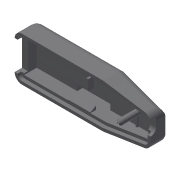
# Autodesk Inventor part: enclbase
Saved by Autodesk Inventor 2022 Beta2 (Build 260130000, 130) ContinuousBuild 0
## iProperties
Shininess: 64.0
Length Units: 11269
Angle Units: 11279
Time Units: 11290
Mass Units: 11283
Length Display Precision: 3
Angle Display Precision: 2
Created: 2002-02-13
Part Number: enclbase
Document SubType Name: Modeling
Designer: Administrator
Density: 1 g/cm^3
Material: Generic
Appearance: Light Gray
Density: 0.0
Volumn: 0.0
Area: 0.0
PropertySet Name: Model Information
Control State: 0
Master: False
Checked Out: False
Last Check In By: PMILLER
Last Check In Date: 2007-04-03
Author: Administrator
Autodesk Inventor part; units mm, degrees
sketch "Sketch1" plane through (0, 0, 0) normal (0, 0, 1) x (1, 0, 0)
  line L0 (8.2169, 11.6469) -> (8.2169, -7.4031)
  line L1 (8.2169, -7.4031) -> (46.3169, -7.4031)
  line L2 (46.3169, -7.4031) -> (66.9544, -4.2281)
  line L3 (66.9544, -4.2281) -> (66.9544, 8.4719)
  line L4 (66.9544, 8.4719) -> (46.3169, 11.6469)
  line L5 (46.3169, 11.6469) -> (8.2169, 11.6469)
  line L6 (66.9544, 2.1219) -> (8.2169, 2.1219) construction
  dimension "d0" = 19.05
  dimension "d1" = 38.1
  dimension "d2" = 58.7375
  dimension "d3" = 12.7
  constraints: 14 end point, 2 equal length, 2 midpoint, 2 parallel, 1 horizontal, 1 perpendicular, 1 vertical
  measures "d0" distance of L0.start L0.end
  measures "d1" distance of L4.end L0.start
  measures "d2" horizontal distance of L3.end L0.start
  measures "d3" distance of L2.end L3.end
extrude "Extrusion1" add sketch "Sketch1" along normal blind 9.525
sketch "Sketch2" plane through (8.2169, -7.4031, 0) normal (0, -1, 0) x (1, 0, 0)
  line L0 (38.1, 0) -> (38.1, 9.525) projected
  line L1 (38.1, 0) -> (58.7375, 0)
  line L2 (58.7375, 0) -> (58.7375, 3.175)
  line L3 (58.7375, 3.175) -> (38.1, 0)
  line L4 (58.7375, 9.525) -> (38.1, 9.525) projected
  line L5 (58.7375, 0) -> (58.7375, 9.525) projected
  dimension "d6" = 6.35
  constraints: 6 end point, 2 perpendicular, 1 collinear
  measures "d6" distance from line of L4 L2.end
extrude "Extrusion2" cut sketch "Sketch2" against normal through all contours L3 L2 L1
shell "Shell1" thickness 2.54 removed faces 1 at (20.9169, -1.0531, 9.525)
sketch "Sketch3" plane through (0, 0, 9.525) normal (0, 0, 1) x (1, 0, 0)
  line L0 (64.4144, 6.2927) -> (64.4144, -2.049) projected
  line L1 (64.4144, -2.049) -> (46.1226, -4.8631) projected
  line L2 (46.1226, -4.8631) -> (10.7569, -4.8631) projected
  line L3 (10.7569, -4.8631) -> (10.7569, 9.1069) projected
  line L4 (10.7569, 9.1069) -> (46.1226, 9.1069) projected
  line L5 (46.1226, 9.1069) -> (64.4144, 6.2927) projected
  line L6 (66.9544, -4.2281) -> (46.3169, -7.4031) projected
  line L7 (66.9544, 8.4719) -> (66.9544, -4.2281) projected
  line L8 (9.4869, 10.3769) -> (46.2197, 10.3769)
  line L9 (46.2197, 10.3769) -> (65.6844, 7.3823)
  line L10 (65.6844, 7.3823) -> (65.6844, -3.1386)
  line L11 (65.6844, -3.1386) -> (46.2197, -6.1331)
  line L12 (46.2197, -6.1331) -> (9.4869, -6.1331)
  line L13 (9.4869, -6.1331) -> (9.4869, 10.3769)
  dimension "d10" = 1.27
  dimension "d11" = 1.27
  dimension "d12" = 1.27
  dimension "d13" = 1.27
  dimension "d14" = 1.27
  constraints: 12 end point, 4 parallel, 3 perpendicular
  measures "d10" horizontal distance of L3.end L8.start
  measures "d11" horizontal distance of L2.end L12.end
  measures "d12" horizontal distance of L9.end L0.start
  measures "d13" distance between parallel lines of L9 L5
  measures "d14" distance from line of L0.end L11
extrude "Extrusion3" cut sketch "Sketch3" against normal blind 1.5875
fillet "Fillet1" radius 3.175 11 edges at (8.2169, 11.6469, 4.7625) (8.2169, -7.4031, 4.7625) (8.2169, 2.1219, 0) (27.2669, -7.4031, 0) (46.3169, -7.4031, 4.7625) (56.6356, -5.8156, 1.5875) (66.9544, -4.2281, 6.35) (27.2669, 11.6469, 0) (46.3169, 11.6469, 4.7625) (56.6356, 10.0594, 1.5875) (66.9544, 8.4719, 6.35)
fillet "Fillet2" radius 1.5875 4 edges at (9.4869, 10.3769, 8.7313) (9.4869, -6.1331, 8.7313) (65.6844, 7.3823, 8.7313) (65.6844, -3.1386, 8.7313)
ref_plane "Work Plane1" through (23.4569, -4.8631, 2.54) normal (1, 0, 0) x (0, 0, -1)
sketch "Sketch4" plane through (66.9544, -1.5043, 9.525) normal (1, 0, 0) x (0, 0, -1)
  line L0 (6.35, 0.4142) -> (6.35, 6.838) projected
  line L1 (2.3812, 8.8028) -> (0, 8.8028)
  line L2 (0, 8.8028) -> (0, 2.4528)
  line L3 (0, 2.4528) -> (0, 2.4528)
  line L4 (2.3812, 4.834) -> (2.3812, 8.8028)
  line L5 (0, -3.1381) -> (3.6261, -3.1381) projected
  line L6 (1.5875, 7.5246) -> (1.5875, -0.2724) projected
  line L7 (0, 7.2522) -> (0, 0) projected
  arc A0 (0, 2.4528) -> (2.3812, 4.834) centre (0, 4.834) ccw
  ellipse E0 centre (3.1376, 6.7638) end of major axis (5.4352, 9.0613) minor radius 3.175 (6.35, 6.838) -> (6.3231, 7.2522) ccw projected
  line L8 (0, 7.2522) -> (6.3231, 7.2522) projected
  line L9 (6.3231, 0) -> (0, 0) projected
  ellipse E1 centre (3.1376, 0.4885) end of major axis (5.4352, -1.8091) minor radius 3.175 (6.3231, 0) -> (6.35, 0.4142) ccw projected
  line L10 (3.6261, 10.3903) -> (0, 10.3903) projected
  point P0 (2.3813, 2.4528)
  dimension "d20" = 6.35
  dimension "d21" = 2.3813
  dimension "d63" = 2.3813
  dimension "d78" = 1.5875
  constraints: 8 end point, 2 perpendicular, 2 point on circle, 2 point on line, 2 tangent, 1 centre point, 1 collinear, 1 parallel, 1 vertical, 2 other
  measures "d20" distance of L1.end L2.end
  measures "d21" distance of L2.end point (2.381, 2.453)
  measures "d63" radius of A0
  measures "d78" distance between parallel lines of L10 L1
extrude "Extrusion4" cut sketch "Sketch4" against normal up to surface (43.4975 mm away) contours L8 L2 L1 L4 | L4 A0 L6 L8 | A0 L2 L8 L6
sketch "Sketch5" plane through (8.2169, -4.2281, 3.175) normal (-1, 0, 0) x (0, 0, 1)
  line L0 (0, 12.7) -> (6.35, 12.7) projected
  line L1 (3.175, 12.7) -> (6.35, 12.7)
  line L2 (6.35, 12.7) -> (6.35, 0)
  line L3 (6.35, 0) -> (3.175, 0)
  line L4 (3.175, 0) -> (3.175, 12.7)
  line L5 (4.7625, -0.3175) -> (4.7625, 13.0175) projected
  line L6 (6.35, 0) -> (6.35, 12.7) projected
  dimension "d26" = 3.175
  constraints: 8 end point, 2 collinear, 2 parallel, 1 horizontal, 1 perpendicular
  measures "d26" distance of L2.end L3.end
extrude "Extrusion5" cut sketch "Sketch5" against normal up to surface (15.24 mm away)
ref_plane "Work Plane2" through (0, 0, 4.7625) normal (0, 0, 1) x (1, 0, 0)
sketch "Sketch6" plane through (0, 0, 4.7625) normal (0, 0, 1) x (1, 0, 0)
  line L0 (55.6831, 7.636) -> (55.6831, -3.3923)
  line L1 (56.4769, 7.5139) -> (56.4769, -3.2702)
  line L2 (64.4144, -2.049) -> (64.4144, 2.5014) projected
  line L3 (57.8767, -3.0548) -> (46.1226, -4.8631) projected
  line L4 (46.1226, 9.1069) -> (64.4144, 6.2927) projected
  line L5 (55.6831, -3.3923) -> (56.4769, -3.2702)
  line L6 (56.4769, 7.5139) -> (55.6831, 7.636)
  dimension "d31" = 0.7937
  dimension "d32" = 7.9375
  constraints: 8 end point, 2 collinear, 1 parallel, 1 vertical
  measures "d31" distance between parallel lines of L1 L0
  measures "d32" distance between parallel lines of L2 L1
extrude "Extrusion6" add sketch "Sketch6" against normal up to next
ref_plane "Work Plane3" through (0, 0, 12.7) normal (0, 0, 1) x (1, 0, 0)
sketch "Sketch7" plane through (0, 0, 12.7) normal (0, 0, 1) x (1, 0, 0)
  circle A0 centre (56.08, 2.1219) radius 1.1906
  circle A1 centre (56.08, 2.1219) radius 5.3897 construction
  circle A2 centre (56.08, 2.1219) radius 0.3969 construction
  line L0 (57.8767, -3.0548) -> (46.1226, -4.8631) projected
  line L1 (46.1226, 9.1069) -> (64.4144, 6.2927) projected
  line L2 (56.4769, -3.2702) -> (56.4769, 7.5139) projected
  line L3 (55.6831, 7.636) -> (55.6831, -3.3923) projected
  dimension "d36" = 2.3813
  constraints: 4 tangent, 3 centre point, 2 coincident
  measures "d36" diameter of A0
extrude "Extrusion7" add sketch "Sketch7" against normal up to surface contours A0 L2 | L2 A0 L3 | L3 A0 surface through (66.5681, -7.4031, 5.6855) normal (-0.1520572, 0, 0.9883717)
sketch "Sketch8" plane through (56.08, 2.1219, 12.7) normal (0, 0, 1) x (1, 0, 0)
  circle A0 centre (0, 0) radius 1.1906 projected
  circle A1 centre (0, 0) radius 0.3969
  dimension "d39" = 0.7937
  constraints: 1 centre point, 1 coincident
  measures "d39" diameter of A1
extrude "Extrusion8" cut sketch "Sketch8" against normal up to surface contours A1 surface through (66.5681, -7.4031, 5.6855) normal (-0.1520572, 0, 0.9883717)
sketch "Sketch10" plane through (10.7569, -4.8631, 2.54) normal (0, 0, 1) x (1, 0, 0)
  line L0 (0, 13.97) -> (0, 0) projected
  line L1 (17.4625, 13.97) -> (31.75, 13.97)
  line L2 (31.75, 13.97) -> (31.75, 11.5887)
  line L3 (17.4625, 11.5887) -> (17.4625, 13.97)
  line L4 (17.4625, 11.5887) -> (31.75, 11.5887)
  dimension "d48" = 2.3813
  dimension "d49" = 14.2875
  dimension "d50" = 17.4625
  constraints: 8 end point, 2 parallel, 1 horizontal, 1 perpendicular
  measures "d48" distance of L3.start L1.start
  measures "d49" distance of L2.end L3.start
  measures "d50" distance from line of L1.start L0
extrude "Extrusion10" cut sketch "Sketch10" against normal up to surface (2.54 mm away)
ref_plane "Work Plane4" through (56.08, 2.1219, 12.7) normal (0, -1, 0) x (1, 0, 0)
chamfer "Chamfer1" distance 0.7937 angle 45 1 edges at (54.8894, 2.1219, 12.7)
ref_plane "Work Plane5" through (34.5694, 6.7256, 2.54) normal (1, 0, 0) x (0, 0, -1)
sketch "Sketch12" plane through (34.5694, 6.7256, 2.54) normal (1, 0, 0) x (0, 0, -1)
  line L0 (-5.3975, 2.3813) -> (-5.3975, 2.1273)
  line L1 (-5.3975, 2.1273) -> (-3.0162, 0.7938)
  line L2 (-3.0162, 0.7938) -> (-3.0162, 2.3813)
  line L3 (-3.0162, 2.3813) -> (-5.3975, 2.3813)
  line L4 (-5.3975, 2.3813) -> (-5.3975, 1.7463) projected
  line L5 (0, 2.3813) -> (-5.3975, 2.3813) projected
  dimension "d67" = 1.5875
  dimension "d68" = 2.3813
  dimension "d69" = 0.254
  constraints: 8 end point, 2 collinear, 1 parallel, 1 perpendicular, 1 vertical
  measures "d67" distance of L1.end L2.end
  measures "d68" distance of L2.end L0.start
  measures "d69" distance of L0.start L0.end
extrude "Extrusion12" add sketch "Sketch12" along normal mid plane 9.525
mirror "Mirror1" about plane through (56.08, 2.1219, 12.7) normal (0, -1, 0) of "Extrusion10", "Extrusion12"
sketch "Sketch13" plane through (46.1226, -4.8631, 2.54) normal (0, 0, 1) x (1, 0, 0)
  line L0 (-3.6158, 11.5887) -> (-17.9033, 11.5888) projected
  line L1 (-17.9033, 11.5888) -> (-17.9033, 13.97) projected
  line L2 (-17.9033, 2.3813) -> (-3.6158, 2.3813) projected
  line L3 (-11.5533, 9.2075) -> (-10.7595, 9.2075)
  line L4 (-10.7595, 9.2075) -> (-10.7595, 4.7625)
  line L5 (-10.7595, 4.7625) -> (-11.5533, 4.7625)
  line L6 (-11.5533, 4.7625) -> (-11.5533, 9.2075)
  dimension "d72" = 0.7937
  dimension "d73" = 2.3813
  dimension "d74" = 2.3813
  dimension "d75" = 6.35
  constraints: 8 end point, 2 parallel, 1 horizontal, 1 perpendicular
  measures "d72" distance of L4.end L5.end
  measures "d73" distance between parallel lines of L0 L3
  measures "d74" distance between parallel lines of L2 L5
  measures "d75" distance between parallel lines of L6 L1
extrude "Extrusion13" add sketch "Sketch13" along normal blind 2.3813
body "Solid1"
